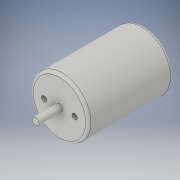
# Autodesk Inventor part: DC Brush Motor 24V 150W High Speed Motor with Belt Pulley for DIY Generator Electric Vehicle Motor
Saved by Autodesk Inventor 2018 (Build 220112000, 112)
## iProperties
Created: 2020-03-23
Part Number: DC Brush Motor 24V 150W High Speed Motor with Belt Pulley for DIY Generator Electric Vehicle Motor
Material: Generic
Document SubType Name: Modeling
Designer: emile
Density: 1 g/cm^3
Appearance: Default
Catalog Web Link: https://www.amazon.ca/dp/B082R32F4K/ref=sspa_dk_detail_2?psc=1&pd_rd_i=B082R32F4K&pd_rd_w=zm4Rm&pf_rd_p=a14ddd24-c45e-4c01-803e-ab6a335c1c48&pd_rd_wg=dEqW1&pf_rd_r=K9WZF461PM65KRFQD8CK&pd_rd_r=499ca0f4-b3ed-4d1e-a3d8-348bb5bb667d&spLa=ZW5jcnlwdGVkUXVhbGlmaWVyPUEzVFVHWU9DWjBTOERaJmVuY3J5cHRlZElkPUEwNzUwMzc1UllIWjk0V1ZITTBQJmVuY3J5cHRlZEFkSWQ9QTAyNDQ0MTAxNUI1UERNWTA4Tlgmd2lkZ2V0TmFtZT1zcF9kZXRhaWwmYWN0aW9uPWNsaWNrUmVkaXJlY3QmZG9Ob3RMb2dDbGljaz10cnVl
Author: emile
Autodesk Inventor part; units mm, degrees
ref_plane "YZ Plane" through (0, 0, 0) normal (1, 0, 0) x (0, 1, 0)
ref_plane "XZ Plane" through (0, 0, 0) normal (0, 1, 0) x (-1, 0, 0)
ref_plane "XY Plane" through (0, 0, 0) normal (0, 0, 1) x (1, 0, 0)
sketch "Sketch1" plane through (0, 0, 0) normal (0, 0, 1) x (1, 0, 0)
  circle A0 centre (0, 0) radius 34
  circle A1 centre (0, 0) radius 4
  circle A2 centre (-18, 0) radius 3.175
  circle A3 centre (18, 0) radius 3.175
  dimension "d0" = 68
  dimension "d1" = 8
  dimension "d2" = 18
  dimension "d3" = 18
  dimension "d4" = 6.35
  constraints: 4 centre point, 2 coincident, 2 horizontal alignment, 1 equal radius
  measures "d0" diameter of A0
  measures "d1" diameter of A1
  measures "d2" distance of A1.centre A3.centre
  measures "d3" distance of A1.centre A2.centre
  measures "d4" diameter of A2
extrude "Extrusion1" add sketch "Sketch1" against normal blind 100 contours A0 | A1 | A2 | A3
extrude "Extrusion2" cut sketch "Sketch1" against normal blind 25.4 contours A2 | A3
extrude "Extrusion3" add sketch "Sketch1" along normal blind 28 contours A1
fillet "Fillet1" radius 3.175 2 edges at (-34, 0, 0) (-34, 0, -100)
equation "\"d3\" = d2"
body "Solid1"
